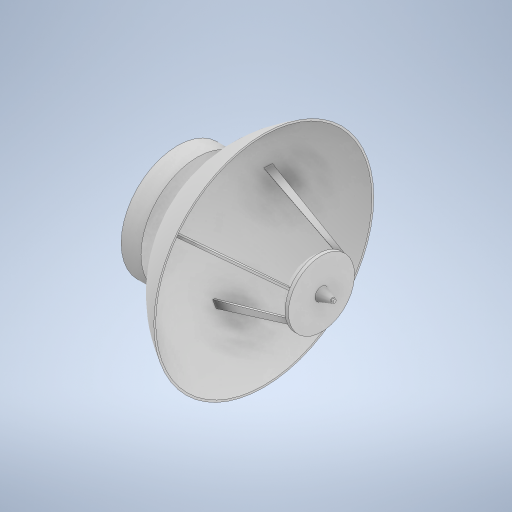
# Autodesk Inventor part: Antenna 23110167
Saved by Autodesk Inventor 2023 (Build 270158000, 158)
## iProperties
Created: 2023-11-11
Part Number: Antenna 23110167
Material: Generic
Document SubType Name: Modeling
Designer: parth
Density: 1 g/cm^3
Appearance: Default
Author: parth
Autodesk Inventor part; units mm, degrees
ref_plane "XZ Plane" through (0, 0, 0) normal (0, 1, 0) x (-1, 0, 0)
ref_plane "XY Plane" through (0, 0, 0) normal (0, 0, 1) x (1, 0, 0)
sketch "Sketch1" plane through (0, 0, 0) normal (0, 0, 1) x (1, 0, 0)
  arc A0 (-1875, 0) -> (-870.2634, -1660.803) centre (0, 0) ccw
  arc A1 (-1850, 0) -> (-870.2634, -1632.5262) centre (0, 0) ccw
  line L0 (-1875, 0) -> (-870.2634, 0)
  line L1 (0, -1850) -> (0, -1875)
  line L2 (-1875, 0) -> (-870.2634, 0)
  line L3 (-870.2634, 0) -> (-870.2634, -1660.803)
  dimension "d0" = 3750
  dimension "d1" = 3700
  constraints: 8 end point, 4 point on circle, 2 centre point, 2 coincident, 2 perpendicular, 2 point on line, 1 horizontal
  measures "d0" diameter of A0
  measures "d1" diameter of A1
revolve "Revolution1" add sketch "Sketch1" angle 360 about axis through (-1875, 0, 0) along (1, 0, 0) contours L0 A1 L3 A0
ref_plane "Work Plane1" through (-1875, 0, 0) normal (1, 0, 0) x (0, 1, 0)
sketch "Sketch2" plane through (-1875, 0, 0) normal (1, 0, 0) x (0, 1, 0)
  circle A0 centre (0, 0) radius 850
  dimension "d3" = 1700
  constraints: 1 centre point, 1 coincident
  measures "d3" diameter of A0
extrude "Extrusion1" add sketch "Sketch2" against normal blind 300
sketch "Sketch3" plane through (0, 0, 0) normal (1, 0, 0) x (0, 1, 0)
  circle A0 centre (0, 0) radius 500
  dimension "d6" = 1000
  constraints: 1 centre point, 1 coincident
  measures "d6" diameter of A0
extrude "Extrusion2" add sketch "Sketch3" against normal blind 50
sketch "Sketch4" plane through (0, 0, 0) normal (0, 0, 1) x (1, 0, 0)
  line L0 (-50, 500) -> (-50, -500) projected
  arc A0 (-50, 500) -> (-50, -500) centre (281.6625, 0) ccw
  line L1 (-50, 0) -> (-318.3375, 0)
  point P0 (0, 0)
  dimension "d9" = 600
  constraints: 3 point on circle, 2 end point, 1 centre point, 1 midpoint
  measures "d9" radius of A0
revolve "Revolution2" add sketch "Sketch4" angle 360 about axis through (-50, 0, 0) along (-1, 0, 0) picked at (-58.9513, -327.0364) contours L0 A0 L1
sketch "Sketch5" plane through (0, 0, 0) normal (0, 0, 1) x (1, 0, 0)
  line L0 (168.8966, 0) -> (0, 0)
  line L1 (0, 0) -> (0, -98.2243)
  line L2 (0, -500) -> (0, 500) projected
  line L3 (168.8966, -38.8364) -> (0, -98.2243)
  line L4 (168.8966, -38.8364) -> (168.8966, 0)
  constraints: 8 end point, 1 horizontal, 1 parallel, 1 point on line
revolve "Revolution3" add sketch "Sketch5" angle 360 about axis through (168.8966, 0, 0) along (-1, 0, 0)
sketch "Sketch6" plane through (168.8966, 0, 0) normal (1, 0, 0) x (0, 0, -1)
  circle A0 centre (0, 0) radius 25
  dimension "d12" = 50
  constraints: 1 centre point, 1 coincident
  measures "d12" diameter of A0
extrude "Extrusion3" add sketch "Sketch6" along normal blind 30
sketch "Sketch7" plane through (0, 0, 0) normal (0, 0, 1) x (1, 0, 0)
  arc A0 (-870.2634, 1632.5262) -> (-870.2634, -1632.5262) centre (0, 0) ccw projected
  line L0 (-50, 500) -> (-50, -500) projected
  line L1 (-1573.9304, -972.2361) -> (-50, -500)
  line L2 (-50, -500) -> (-50, -453.825)
  arc A1 (-50, 500) -> (-50, -500) centre (281.6625, 0) ccw projected
  line L3 (-110.8204, -453.825) -> (-1626.066, -882.275)
  arc A2 (-870.2634, 1632.5262) -> (-870.2634, -1632.5262) centre (0, 0) ccw projected
  arc A3 (-110.8204, -453.825) -> (-50, -500) centre (281.6625, 0) ccw
  arc A4 (-1626.066, -882.275) -> (-1573.9304, -972.2361) centre (0, 0) ccw
  constraints: 7 point on circle, 6 end point, 2 centre point, 2 concentric, 1 point on line
extrude "Extrusion4" add sketch "Sketch7" along normal mid plane 30 contours L3 A1 L1 A0
pattern_circular "Circular Pattern1" count 3 over 360 about axis through (0, 0, 0) along (-1, 0, 0) of "Extrusion4"
body "Solid1"
